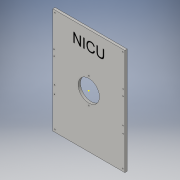
# Autodesk Inventor part: FrontplatteII
Saved by Autodesk Inventor 2016 (Build 200138000, 138)
## iProperties
Created: 2016-06-13
Part Number: FrontplatteII
Material: Generic
Document SubType Name: Modeling
Designer: Ju
Density: 1 g/cm^3
Appearance: Default
Author: Ju
Autodesk Inventor part; units mm, degrees
ref_plane "YZ Plane" through (0, 0, 0) normal (1, 0, 0) x (0, 1, 0)
ref_plane "XZ Plane" through (0, 0, 0) normal (0, 1, 0) x (-1, 0, 0)
ref_plane "XY Plane" through (0, 0, 0) normal (0, 0, 1) x (1, 0, 0)
sketch "Sketch1" plane through (0, 0, 0) normal (0, 0, 1) x (1, 0, 0)
  line L0 (75, 110) -> (-75, 110)
  line L1 (-75, 110) -> (-75, -110)
  line L2 (-75, -110) -> (75, -110)
  line L3 (75, -110) -> (75, 110)
  circle A0 centre (0, 0) radius 22.25
  circle A1 centre (0, -26.75) radius 1
  circle A2 centre (0, 26.75) radius 1
  circle A3 centre (108.4721, 5.5003) radius 1.5
  circle A4 centre (70.5, 105) radius 1
  circle A5 centre (-70.5, 105) radius 1
  circle A6 centre (70.5, -105) radius 1
  circle A7 centre (-70.5, -105) radius 1
  dimension "d0" = 150
  dimension "d1" = 220
  dimension "d2" = 44.5
  dimension "d3" = 2
  dimension "d4" = 2
  dimension "d5" = 3
  dimension "d6" = 2
  dimension "d7" = 2
  dimension "d8" = 2
  dimension "d9" = 2
  constraints: 8 centre point, 8 end point, 2 parallel, 1 coincident, 1 horizontal, 1 perpendicular
  measures "d0" distance of L2.end L1.end
  measures "d1" distance of L1.end L0.end
  measures "d2" diameter of A0
  measures "d3" diameter of A1
  measures "d4" diameter of A2
  measures "d5" diameter of A3
  measures "d6" diameter of A4
  measures "d7" diameter of A5
  measures "d8" diameter of A6
  measures "d9" diameter of A7
extrude "Extrusion1" add sketch "Sketch1" along normal blind 5 contours L3 L2 L1 L0
sketch "Sketch2" plane through (0, 0, 5) normal (0, 0, 1) x (1, 0, 0)
  line L0 (-34.154, 91.1798) -> (34.154, 91.1798) construction
  line L1 (34.154, 91.1798) -> (34.154, 70.4938) construction
  line L2 (34.154, 70.4938) -> (-34.154, 70.4938) construction
  line L3 (-34.154, 70.4938) -> (-34.154, 91.1798) construction
  point P0 (0, 0)
  constraints: 2 other
hole "Hole1" at (71.2413, 25.6886, 5) direction (0, 0, -1) diameter 2 end through all
hole "Hole2" at (-71.9717, 26.0836, 5) direction (0, 0, -1) diameter 2 end through all
hole "Hole3" at (-72.3668, 38.3308, 5) direction (0, 0, -1) diameter 2 end through all
hole "Hole4" at (71.4388, 38.7259, 5) direction (0, 0, -1) diameter 2 end through all
hole "Hole5" at (-71.1816, -25.2755, 5) direction (0, 0, -1) diameter 2 end through all
hole "Hole6" at (71.2413, -27.0533, 5) direction (0, 0, -1) diameter 2 end through all
hole "Hole7" at (71.4388, -41.6709, 5) direction (0, 0, -1) diameter 2 end through all
hole "Hole8" at (-71.3791, -42.2635, 5) direction (0, 0, -1) diameter 2 end through all
body "Solid1"
